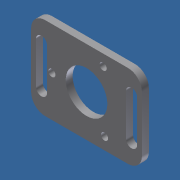
# Autodesk Inventor part: dewalt tom mounting plate
Saved by Autodesk Inventor 2012 (Build 160160000, 160)
## iProperties
Created: 2012-07-12
Part Number: dewalt tom mounting plate
Material: Default
Document SubType Name: Modeling
Designer: Team-2471
Density: 1 g/cm^3
Author: Team-2471
Autodesk Inventor part; units mm, degrees
ref_plane "YZ Plane" through (0, 0, 0) normal (1, 0, 0) x (0, 1, 0)
ref_plane "XZ Plane" through (0, 0, 0) normal (0, 1, 0) x (-1, 0, 0)
ref_plane "XY Plane" through (0, 0, 0) normal (0, 0, 1) x (1, 0, 0)
sketch "Sketch1" plane through (0, 0, 0) normal (0, 0, 1) x (1, 0, 0)
  line L0 (-28.575, 19.05) -> (28.575, 19.05)
  line L1 (28.575, 19.05) -> (28.575, -19.05)
  line L2 (28.575, -19.05) -> (-28.575, -19.05)
  line L3 (-28.575, -19.05) -> (-28.575, 19.05)
  circle A0 centre (0, 0) radius 9.525
  circle A1 centre (0, 0) radius 15.875
  line L4 (-26.3525, 9.525) -> (-21.2725, 9.525)
  line L5 (-21.2725, 9.525) -> (-21.2725, -9.525)
  line L6 (-21.2725, -9.525) -> (-26.3525, -9.525)
  line L7 (-26.3525, -9.525) -> (-26.3525, 9.525)
  arc A2 (-21.2725, 9.525) -> (-26.3525, 9.525) centre (-23.8125, 9.525) ccw
  arc A3 (-26.3525, -9.525) -> (-21.2725, -9.525) centre (-23.8125, -9.525) ccw
  line L8 (21.2725, 9.525) -> (26.3525, 9.525)
  line L9 (26.3525, 9.525) -> (26.3525, -9.525)
  line L10 (26.3525, -9.525) -> (21.2725, -9.525)
  line L11 (21.2725, -9.525) -> (21.2725, 9.525)
  arc A4 (26.3525, 9.525) -> (21.2725, 9.525) centre (23.8125, 9.525) ccw
  arc A5 (21.2725, -9.525) -> (26.3525, -9.525) centre (23.8125, -9.525) ccw
  point P0 (7.6157, 13.929)
  point P1 (-15.8707, -0.3691)
  point P2 (8.255, -13.5599)
  dimension "d5" = 31.75
  dimension "d0" = 19.05
  dimension "d1" = 19.05
  dimension "d2" = 38.1
  dimension "d3" = 28.575
  dimension "d4" = 57.15
  dimension "d8" = 360
  dimension "d11" = 4.7625
  dimension "d12" = 19.05
  dimension "d13" = 9.525
  dimension "d14" = 5.08
  dimension "d15" = 19.05
  dimension "d16" = 5.08
  dimension "d17" = 4.7625
  dimension "d33" = 8.255
  constraints: 24 end point, 8 point on circle, 8 tangent, 6 parallel, 5 centre point, 3 horizontal, 3 perpendicular, 2 coincident, 1 collinear, 7 other
  measures "d0" diameter of A0
  measures "d1" distance from line of L0 point (0, 0)
  measures "d2" distance of L0.end L1.end
  measures "d3" distance from line of L3 point (0, 0)
  measures "d4" distance of L0.start L0.end
  measures "d11" distance from line of L3 A2.centre
  measures "d12" distance of L6.end L4.start
  measures "d13" distance between parallel lines of L4 L0
  measures "d14" distance between parallel lines of L5 L7
  measures "d15" distance of L10.end L11.end
  measures "d16" distance between parallel lines of L9 L11
  measures "d17" distance from line of L1 A4.centre
  measures "d33" horizontal distance of point (8.255, -13.56) point (0, 0)
extrude "Extrusion1" add sketch "Sketch1" against normal blind 3.175 contours L0 L1 L2 L3 | A1
hole "Hole1" at (7.6157, 13.929, 0) at (-15.8707, -0.3691, 0) at (8.255, -13.5599, 0) direction (0, 0, -1) diameter 3.2512 end through all
fillet "Fillet1" radius 6.35 4 edges at (28.575, 19.05, -1.5875) (-28.575, 19.05, -1.5875) (-28.575, -19.05, -1.5875) (28.575, -19.05, -1.5875)
equation "\"d4\" = 2 * d3"
equation "\"d17\" = d11"
body "Solid1"
